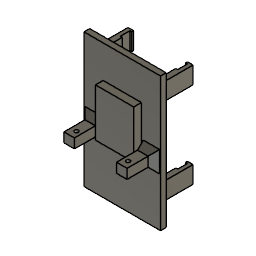
Wrist2 (Autodesk Fusion 360 design; units mm, degrees)
Autodesk Fusion 360 part; units mm, degrees
sketch "Sketch1" plane through (0, 0, 0) normal (0, 1, 0) x (1, 0, 0)
  line L0 (-20, -35) -> (20, -35)
  line L1 (20, -35) -> (20, 35)
  line L2 (20, 35) -> (-20, 35)
  line L3 (-20, 35) -> (-20, -35)
  line L4 (-14.65, -4.5) -> (-12.65, -4.5)
  line L5 (-12.65, -4.5) -> (-12.65, 4.5)
  line L6 (-12.65, 4.5) -> (-14.65, 4.5)
  line L7 (-14.65, 4.5) -> (-14.65, -4.5)
  line L8 (12.65, -4.5) -> (14.65, -4.5)
  line L9 (14.65, -4.5) -> (14.65, 4.5)
  line L10 (14.65, 4.5) -> (12.65, 4.5)
  line L11 (12.65, 4.5) -> (12.65, -4.5)
  line L12 (-12.65, -4.5) -> (-11.65, -4.5)
  line L13 (-11.65, -4.5) -> (-11.65, 4.5)
  line L14 (-11.65, 4.5) -> (-12.65, 4.5)
  line L15 (-12.65, 4.5) -> (-12.65, -4.5)
  line L16 (12.65, -4.5) -> (11.65, -4.5)
  line L17 (11.65, -4.5) -> (11.65, 4.5)
  line L18 (11.65, 4.5) -> (12.65, 4.5)
  line L19 (12.65, 4.5) -> (12.65, -4.5)
  circle A0 centre (0, 0) radius 5
  line L20 (14, 16.5) -> (14, 25.5)
  line L21 (15, 16.5) -> (14, 16.5)
  line L22 (17, 16.5) -> (17, 25.5)
  line L23 (15, 25.5) -> (15, 16.5)
  line L24 (15, 16.5) -> (17, 16.5)
  line L25 (15, 25.5) -> (15, 16.5)
  line L26 (15, -19.5) -> (15, -28.5)
  line L27 (15, -19.5) -> (15, -28.5)
  line L28 (15, -28.5) -> (17, -28.5)
  line L29 (14, -28.5) -> (14, -19.5)
  line L30 (15, -28.5) -> (14, -28.5)
  line L31 (17, -28.5) -> (17, -19.5)
  line L32 (-15, -28.5) -> (-15, -19.5)
  line L33 (-17, -19.5) -> (-17, -28.5)
  line L34 (-15, -28.5) -> (-14, -28.5)
  line L35 (-14, -28.5) -> (-14, -19.5)
  line L36 (-15, -19.5) -> (-17, -19.5)
  line L37 (-15, -19.5) -> (-15, -28.5)
  line L38 (-14, -19.5) -> (-15, -19.5)
  line L39 (-17, -28.5) -> (-15, -28.5)
  line L40 (-15, 16.5) -> (-15, 25.5)
  line L41 (-17, 25.5) -> (-17, 16.5)
  line L42 (-15, 16.5) -> (-14, 16.5)
  line L43 (-14, 16.5) -> (-14, 25.5)
  line L44 (-15, 25.5) -> (-17, 25.5)
  line L45 (-15, 25.5) -> (-15, 16.5)
  line L46 (-14, 25.5) -> (-15, 25.5)
  line L47 (-17, 16.5) -> (-15, 16.5)
  line L48 (17, 25.5) -> (14, 25.5)
  line L49 (17, -19.5) -> (14, -19.5)
  line L50 (12.65, 1.5) -> (14.65, 1.5)
  line L51 (-14.65, 1.5) -> (-12.65, 1.5)
  line L52 (-10, -18) -> (10, -18)
  line L53 (10, -18) -> (10, 7)
  line L54 (10, 7) -> (-10, 7)
  line L55 (-10, 7) -> (-10, -18)
  line L56 (16.5, 1.5) -> (10.5, 1.5)
  line L57 (10.5, 1.5) -> (10.5, 6.5)
  line L58 (10.5, 6.5) -> (16.5, 6.5)
  line L59 (16.5, 6.5) -> (16.5, 1.5)
  line L60 (-10.5, 1.5) -> (-16.5, 1.5)
  line L61 (-16.5, 1.5) -> (-16.5, 6.5)
  line L62 (-16.5, 6.5) -> (-10.5, 6.5)
  line L63 (-10.5, 6.5) -> (-10.5, 1.5)
  dimension "d1" = 40
  dimension "d2" = 70
  dimension "d3" = 20
  dimension "d4" = 35
  dimension "d5" = 9
  dimension "d6" = 2
  dimension "d7" = 4.5
  dimension "d8" = 12.65
  dimension "d9" = 2
  dimension "d10" = 9
  dimension "d11" = 12.65
  dimension "d12" = 4.5
  dimension "d13" = 1
  dimension "d14" = 9
  dimension "d15" = 1
  dimension "d16" = 9
  dimension "d17" = 10
  dimension "d18" = 2
  dimension "d19" = 9
  dimension "d20" = 1
  dimension "d21" = 9
  dimension "d22" = 2
  dimension "d23" = 9
  dimension "d24" = 1
  dimension "d25" = 9
  dimension "d26" = 9
  dimension "d27" = 2
  dimension "d28" = 1
  dimension "d29" = 9
  dimension "d30" = 9
  dimension "d31" = 2
  dimension "d32" = 1
  dimension "d33" = 9
  dimension "d40" = 3
  dimension "d41" = 3
  dimension "d58" = 20
  dimension "d59" = 25
  dimension "d60" = 10
  dimension "d61" = 18
  dimension "d64" = 6
  dimension "d65" = 5
  dimension "d66" = 2.15
  dimension "d67" = 2.15
  dimension "d79" = 3
  dimension "d80" = 3
  dimension "d81" = 3
  dimension "d82" = 3
  constraint horizontal L0
  constraint vertical L1
  constraint horizontal L2
  constraint vertical L3
  constraint horizontal L4
  constraint vertical L5
  constraint horizontal L6
  constraint vertical L7
  constraint horizontal L8
  constraint vertical L9
  constraint horizontal L10
  constraint vertical L11
  constraint horizontal L12
  constraint vertical L13
  constraint horizontal L14
  constraint vertical L15
  constraint horizontal L16
  constraint vertical L17
  constraint horizontal L18
  constraint vertical L19
  constraint coincident A0.centre origin
  constraint horizontal L24
  constraint vertical L22
  constraint vertical L25
  constraint horizontal L21
  constraint vertical L20
  constraint vertical L23
  constraint horizontal L28
  constraint vertical L31
  constraint vertical L27
  constraint horizontal L30
  constraint vertical L29
  constraint vertical L26
  constraint horizontal L39
  constraint vertical L32
  constraint horizontal L36
  constraint vertical L33
  constraint horizontal L34
  constraint vertical L35
  constraint horizontal L38
  constraint vertical L37
  constraint horizontal L47
  constraint vertical L40
  constraint horizontal L44
  constraint vertical L41
  constraint horizontal L42
  constraint vertical L43
  constraint horizontal L46
  constraint vertical L45
  constraint perpendicular L20 L48
  constraint perpendicular L29 L49
  constraint coincident L11 L50.start
  constraint coincident L9 L50.end
  constraint perpendicular L9 L50
  constraint coincident L7 L51.start
  constraint coincident L5 L51.end
  constraint perpendicular L5 L51
  constraint horizontal L52
  constraint vertical L53
  constraint horizontal L54
  constraint vertical L55
  constraint horizontal L56
  constraint vertical L57
  constraint horizontal L58
  constraint vertical L59
  constraint horizontal L60
  constraint vertical L61
  constraint horizontal L62
  constraint vertical L63
  measures "d1" distance of L0.start L0.end
  measures "d2" distance of L0.start L2.end
  measures "d3" horizontal distance of A0.centre L0.start
  measures "d4" vertical distance of A0.centre L0.start
  measures "d5" distance of L4.start L6.end
  measures "d6" distance of L5.end L6.end
  measures "d7" vertical distance of A0.centre L4.end
  measures "d8" distance of A0.centre L5
  measures "d9" distance of L8.start L8.end
  measures "d10" distance of L8.start L10.end
  measures "d11" distance of A0.centre L11
  measures "d12" vertical distance of A0.centre L10.end
  measures "d13" distance of L4.end L12.end
  measures "d14" distance of L4.end L5.end
  measures "d15" distance of L8.start L16.end
  measures "d16" distance of L8.start L10.end
  measures "d17" diameter of A0
  measures "d18" distance of L22.start L21.start
  measures "d19" distance of L21.start L23.start
  measures "d20" distance of L21.start L20.start
  measures "d21" distance of L23.start L21.start
  measures "d22" distance of L28.end L26.end
  measures "d23" distance of L26.start L26.end
  measures "d24" distance of L26.end L29.start
  measures "d25" distance of L26.end L26.start
  measures "d26" distance of L33.end L33.start
  measures "d27" distance of L32.end L33.start
  measures "d28" distance of L32.start L34.end
  measures "d29" distance of L32.start L32.end
  measures "d30" distance of L41.end L41.start
  measures "d31" distance of L40.end L41.start
  measures "d32" distance of L40.start L42.end
  measures "d33" distance of L40.start L40.end
  measures "d40" distance of L10.end L50.start
  measures "d41" distance of L6.end L51.start
  measures "d58" distance of L52.start L52.end
  measures "d59" distance of L52.start L54.end
  measures "d60" distance of A0.centre L55
  measures "d61" distance of A0.centre L52
  measures "d64" distance of L60.start L60.end
  measures "d65" distance of L60.start L62.end
  measures "d66" distance of L19 L57
  measures "d67" distance of L5 L63
  measures "d79" distance of L1 L31
  measures "d80" distance of L3 L33
  measures "d81" distance of L1 L22
  measures "d82" distance of L3 L41
extrude "Extrude1" add sketch "Sketch1" along normal blind 3 contours L0 L1 L2 L3 | L4 L5 L7 L15 L51 L60 | L5 L12 L13 L15 L60 | L6 L7 L13 L14 L60 L61 L62 L63 | L5 L6 L7 L15 L51 L60 | L5 L13 L14 L15 L60 | L8 L9 L11 L19 L50 L56 | L11 L16 L17 L19 L56 | L11 L17 L18 L19 L56 | L9 L10 L11 L19 L50 L56 | L9 L10 L17 L18 L56 L57 L58 L59 | A0 | L20 L21 L23 L25 L48 | L22 L23 L24 L25 L48 | L26 L27 L28 L31 L49 | L26 L27 L29 L30 L49 | L32 L33 L36 L37 L39 | L32 L34 L35 L37 L38 | L40 L41 L44 L45 L47 | L40 L42 L43 L45 L46 | L52 L53 L54 L55
extrude "Extrude2" add sketch "Sketch1" against normal blind 14 contours L6 L7 L13 L14 L60 L61 L62 L63 | L5 L6 L7 L15 L51 L60 | L5 L13 L14 L15 L60 | L11 L17 L18 L19 L56 | L9 L10 L11 L19 L50 L56 | L9 L10 L17 L18 L56 L57 L58 L59
extrude "Extrude4" add sketch "Sketch1" along normal blind 20 contours L20 L21 L23 L25 L48 | L22 L23 L24 L25 L48 | L26 L27 L28 L31 L49 | L26 L27 L29 L30 L49 | L32 L33 L36 L37 L39 | L32 L34 L35 L37 L38 | L40 L41 L44 L45 L47 | L40 L42 L43 L45 L46
extrude "Extrude5" cut sketch "Sketch1" along normal blind 19 contours L20 L21 L23 L25 L48 | L26 L27 L29 L30 L49 | L32 L34 L35 L37 L38 | L40 L42 L43 L45 L46
extrude "Extrude6" add sketch "Sketch1" along normal blind 14 contours L20 L21 L23 L25 L48 | L26 L27 L29 L30 L49 | L32 L34 L35 L37 L38 | L40 L42 L43 L45 L46
chamfer "Chamfer3" distance 2 angle 45 12 edges at (-15.5, 3, -16.5) (-17, 3, 24) (-17, 3, -21) (-15.5, 3, -25.5) (15.5, 3, -25.5) (17, 3, -21) (15.5, 3, -16.5) (15.5, 3, 19.5) (17, 3, 24) (15.5, 3, 28.5) (-15.5, 3, 28.5) (-15.5, 3, 19.5)
extrude "Extrude7" add sketch "Sketch1" against normal blind 4 contours A0 | L52 L53 L54 L55
sketch "Sketch2" plane through (0, 0, -1.5) normal (0, 0, 1) x (-1, 0, 0)
  line L0 (10.5, 0) -> (16.5, 0)
  line L1 (16.5, 0) -> (16.5, 14)
  line L2 (16.5, 14) -> (10.5, 14)
  line L3 (10.5, 14) -> (10.5, 0)
  circle A0 centre (13.5, 10.39) radius 1
  circle A1 centre (-13.5, 10.39) radius 1
  line L4 (-10.5, 0) -> (-10.5, 14)
  line L5 (20, 0) -> (-20, 0)
  dimension "d68" = 2
  dimension "d70" = 10.39
  dimension "d71" = 3
  dimension "d72" = 2
  dimension "d73" = 3
  dimension "d74" = 10.39
  measures "d68" diameter of A0
  measures "d70" distance of L0 A0.centre
  measures "d71" distance of L3 A0.centre
  measures "d72" diameter of A1
  measures "d73" distance of A1.centre L4
  measures "d74" distance of A1.centre L5
extrude "Extrude8" cut sketch "Sketch2" against normal blind 9 contours A0 | A1
chamfer "Chamfer4" distance 3 angle 45 6 edges at (16.5, 0, -4) (13.5, 0, -1.5) (13.5, 0, -6.5) (-13.5, 0, -6.5) (-16.5, 0, -4) (-13.5, 0, -1.5)
move_face "OffsetFaces1" offset -0.5 2 faces at (10.5, -6.6667, -4.8333) (-10.5, -6.6667, -3.1667)
